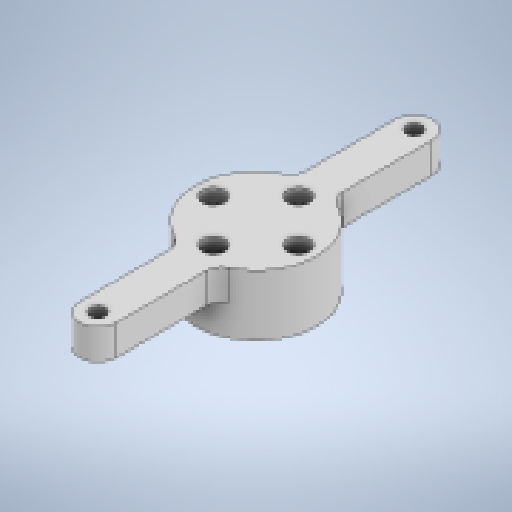
# Autodesk Inventor part: gripper_base_frame
Saved by Autodesk Inventor 2024 (Build 280153000, 153)
## iProperties
Created: 2023-09-01
Part Number: gripper_base_frame
Material: 일반
Document SubType Name: Modeling
Designer: 박동준
Density: 1 g/cm^3
Appearance: 기본값
Author: 박동준
Autodesk Inventor part; units mm, degrees
ref_plane "YZ Plane" through (0, 0, 0) normal (1, 0, 0) x (0, 1, 0)
ref_plane "XZ Plane" through (0, 0, 0) normal (0, 1, 0) x (-1, 0, 0)
ref_plane "XY Plane" through (0, 0, 0) normal (0, 0, 1) x (1, 0, 0)
sketch "스케치1" plane through (0, 0, 0) normal (0, 1, 0) x (-1, 0, 0)
  circle A0 centre (0, 0) radius 10
  dimension "d0" = 20
  constraints: 1 centre point, 1 coincident
  measures "d0" diameter of A0
extrude "돌출1" add sketch "스케치1" along normal blind 10
sketch "스케치2" plane through (0, 10, 0) normal (0, 1, 0) x (1, 0, 0)
  circle A0 centre (0, 0) radius 7
  point P0 (0, 7)
  point P1 (-7, 0)
  point P2 (0, -7)
  point P3 (7, 0)
  dimension "d3" = 14
  constraints: 4 point on circle, 2 horizontal alignment, 2 vertical alignment, 1 centre point, 1 coincident
  measures "d3" diameter of A0
hole "구멍1" at (0, 10, -7) at (-7, 10, 0) at (0, 10, 7) at (7, 10, 0) direction (0, -1, 0) diameter 2.1 end through all counterbore diameter 3.7 counterbore depth 2.2
sketch "스케치3" plane through (0, 10, 0) normal (0, 1, 0) x (1, 0, 0)
  circle A0 centre (0, -7) radius 1.85 projected
  circle A1 centre (0, 7) radius 1.85 projected
  circle A2 centre (-7, 0) radius 1.85 projected
  circle A3 centre (7, 0) radius 1.85 projected
  circle A4 centre (0, 0) radius 10 projected
  circle A5 centre (0, 26) radius 2
  circle A6 centre (0, -26) radius 2
  arc A7 (3, 26) -> (-3, 26) centre (0, 26) ccw
  line L0 (-3, 26) -> (-3, 11.225)
  circle A8 centre (0, 0) radius 10 projected
  line L1 (3, 26) -> (3, 11.225)
  circle A9 centre (0, 0) radius 10
  arc A10 (-4.4, 8.98) -> (-3, 11.225) centre (-5.5, 11.225) ccw
  circle A11 centre (0, 0) radius 10 projected
  line L2 (-5.5, 11.225) -> (-4.4, 8.98) construction
  line L3 (-5.5, 11.225) -> (-3, 11.225) construction
  line L4 (0, 7) -> (0, 26)
  line L5 (3, 26) -> (3, 11.225)
  arc A12 (3, 11.225) -> (4.4, 8.98) centre (5.5, 11.225) ccw
  circle A13 centre (7, 0) radius 1.05 projected
  line L6 (-7, 0) -> (7, 0) construction
  circle A14 centre (0, -26) radius 2
  arc A15 (-3, -26) -> (3, -26) centre (0, -26) ccw
  line L7 (-3, -26) -> (-3, -11.225)
  line L8 (3, -26) -> (3, -11.225)
  arc A16 (-3, -11.225) -> (-4.4, -8.98) centre (-5.5, -11.225) ccw
  arc A17 (4.4, -8.98) -> (3, -11.225) centre (5.5, -11.225) ccw
  dimension "d11" = 4
  dimension "d12" = 4
  dimension "d13" = 26
  dimension "d14" = 26
  dimension "d15" = 3
  dimension "d19" = 5
  dimension "d20" = 3
  constraints: 18 end point, 13 symmetric about line, 12 point on circle, 10 centre point, 3 coincident, 2 tangent, 2 vertical, 2 vertical alignment, 1 concentric, 1 horizontal, 8 other
  measures "d11" diameter of A5
  measures "d12" diameter of A6
  measures "d13" distance of A5.centre point (0, 0)
  measures "d14" distance of A6.centre point (0, 0)
  measures "d15" radius of A7
  measures "d19" diameter of A10
  measures "d20" distance from line of L0 A5.centre
extrude "돌출2" add sketch "스케치3" against normal blind 5 contours A4 A10 L0 A7 L1 A12 | A17 L8 A15 L7 A16 A4 | A5 | A6
sketch "스케치4" plane through (0, 10, 0) normal (0, 1, 0) x (1, 0, 0)
  circle A0 centre (0, -7) radius 1.85 projected
  circle A1 centre (0, 7) radius 1.85 projected
  circle A2 centre (-7, 0) radius 1.85 projected
  circle A3 centre (7, 0) radius 1.85 projected
  arc A4 (-4.4, 8.98) -> (-4.4, -8.98) centre (0, 0) ccw projected
  arc A5 (-3, -11.225) -> (-4.4, -8.98) centre (-5.5, -11.225) ccw projected
  line L0 (-3, -11.225) -> (-3, -26) projected
  arc A6 (-3, -26) -> (3, -26) centre (0, -26) ccw projected
  line L1 (3, -26) -> (3, -11.225) projected
  arc A7 (4.4, -8.98) -> (3, -11.225) centre (5.5, -11.225) ccw projected
  arc A8 (4.4, -8.98) -> (4.4, 8.98) centre (0, 0) ccw projected
  arc A9 (3, 11.225) -> (4.4, 8.98) centre (5.5, 11.225) ccw projected
  line L2 (3, 11.225) -> (3, 26) projected
  arc A10 (3, 26) -> (-3, 26) centre (0, 26) ccw projected
  line L3 (-3, 26) -> (-3, 11.225) projected
  arc A11 (-4.4, 8.98) -> (-3, 11.225) centre (-5.5, 11.225) ccw projected
  constraints: 4 coincident
hole "구멍2" at (0, 10, -26) at (0, 10, 26) direction (0, -1, 0) diameter 2.459 end through all thread size "M3x0.5" class "6H" standard "ISO Metric profile"
